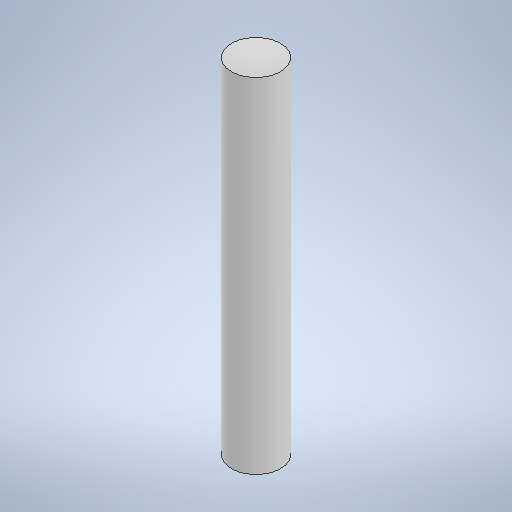
# Autodesk Inventor part: 45-02-004
Saved by Autodesk Inventor 2025.2 (Build 292293000, 293)
## iProperties
Created: 2024-11-14
Part Number: 45-02-004
Material: Generic
Document SubType Name: Modeling
Designer: Zvonko.Gabric
Density: 1 g/cm^3
Appearance: Default
Author: Zvonko.Gabric
Autodesk Inventor part; units mm, degrees
ref_plane "YZ Plane" through (0, 0, 0) normal (1, 0, 0) x (0, 1, 0)
ref_plane "XZ Plane" through (0, 0, 0) normal (0, 1, 0) x (-1, 0, 0)
ref_plane "XY Plane" through (0, 0, 0) normal (0, 0, 1) x (1, 0, 0)
sketch "Sketch2" plane through (0, 0, 0) normal (0, 1, 0) x (-1, 0, 0)
  circle A0 centre (0, 0) radius 2
  dimension "d42" = 4
  constraints: 1 centre point, 1 coincident
  measures "d42" diameter of A0
extrude "Extrusion1" add sketch "Sketch2" along normal blind 28
sketch "Sketch5" plane through (0, 0, 0) normal (1, 0, 0) x (0, 1, 0)
  line L0 (0, 0) -> (-0.57, 0)
  line L1 (0, -2) -> (0, 2) projected
  arc A0 (-0.57, 0) -> (0, -2) centre (2.929, -0.084) ccw
  dimension "d43" = 0.57
  dimension "d48" = 3.5
  constraints: 2 end point, 2 point on circle, 1 centre point, 1 horizontal
  measures "d43" distance of L0.start L0.end
  measures "d48" radius of A0
revolve "Revolution1" add sketch "Sketch5" angle 360 about axis through (0, 0, 0) along (0, -1, 0)
sketch "Sketch6" plane through (0, 0, 0) normal (1, 0, 0) x (0, 1, 0)
  line L0 (28, -2) -> (28, 2) projected
  line L1 (28, 0) -> (28.57, 0)
  arc A0 (28, -2) -> (28.57, 0) centre (25.071, -0.084) ccw
  point P0 (0, 0)
  dimension "d49" = 3.5
  dimension "d50" = 0.57
  constraints: 2 end point, 2 point on circle, 1 centre point, 1 horizontal, 1 midpoint
  measures "d49" radius of A0
  measures "d50" distance of L1.start L1.end
revolve "Revolution2" add sketch "Sketch6" angle 360 about axis through (0, 28, 0) along (0, 1, 0)
body "Solid1"
